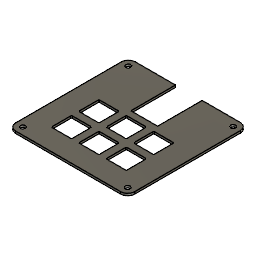
SpeedrunDeck+front (Autodesk Fusion 360 design; units mm, degrees)
part number: 2025-12-30-22-12-29-423
Autodesk Fusion 360 part; units mm, degrees
sketch "plate-2025-12-30T20_28_05.150Z" plane through (0, 0, 0) normal (0, 0, 1) x (1, 0, 0)
  line L0 (5.2708, 37.2959) -> (18.2708, 37.2959)
  line L1 (5.2708, 23.2959) -> (18.2708, 23.2959)
  line L2 (4.7708, 36.7959) -> (4.7708, 23.7959)
  line L3 (18.7708, 36.7959) -> (18.7708, 23.7959)
  arc A0 (5.2708, 37.2959) -> (4.7708, 36.7959) centre (5.2708, 36.7959) ccw
  arc A1 (18.7708, 36.7959) -> (18.2708, 37.2959) centre (18.2708, 36.7959) ccw
  arc A2 (4.7708, 23.7959) -> (5.2708, 23.2959) centre (5.2708, 23.7959) ccw
  arc A3 (18.2708, 23.2959) -> (18.7708, 23.7959) centre (18.2708, 23.7959) ccw
  line L4 (24.3208, 37.2959) -> (37.3208, 37.2959)
  line L5 (24.3208, 23.2959) -> (37.3208, 23.2959)
  line L6 (23.8208, 36.7959) -> (23.8208, 23.7959)
  line L7 (37.8208, 36.7959) -> (37.8208, 23.7959)
  arc A4 (24.3208, 37.2959) -> (23.8208, 36.7959) centre (24.3208, 36.7959) ccw
  arc A5 (37.8208, 36.7959) -> (37.3208, 37.2959) centre (37.3208, 36.7959) ccw
  arc A6 (23.8208, 23.7959) -> (24.3208, 23.2959) centre (24.3208, 23.7959) ccw
  arc A7 (37.3208, 23.2959) -> (37.8208, 23.7959) centre (37.3208, 23.7959) ccw
  line L8 (43.3708, 37.2959) -> (56.3708, 37.2959)
  line L9 (43.3708, 23.2959) -> (56.3708, 23.2959)
  line L10 (42.8708, 36.7959) -> (42.8708, 23.7959)
  line L11 (56.8708, 36.7959) -> (56.8708, 23.7959)
  arc A8 (43.3708, 37.2959) -> (42.8708, 36.7959) centre (43.3708, 36.7959) ccw
  arc A9 (56.8708, 36.7959) -> (56.3708, 37.2959) centre (56.3708, 36.7959) ccw
  arc A10 (42.8708, 23.7959) -> (43.3708, 23.2959) centre (43.3708, 23.7959) ccw
  arc A11 (56.3708, 23.2959) -> (56.8708, 23.7959) centre (56.3708, 23.7959) ccw
  line L12 (5.2708, 18.2459) -> (18.2708, 18.2459)
  line L13 (5.2708, 4.2459) -> (18.2708, 4.2459)
  line L14 (4.7708, 17.7459) -> (4.7708, 4.7459)
  line L15 (18.7708, 17.7459) -> (18.7708, 4.7459)
  arc A12 (5.2708, 18.2459) -> (4.7708, 17.7459) centre (5.2708, 17.7459) ccw
  arc A13 (18.7708, 17.7459) -> (18.2708, 18.2459) centre (18.2708, 17.7459) ccw
  arc A14 (4.7708, 4.7459) -> (5.2708, 4.2459) centre (5.2708, 4.7459) ccw
  arc A15 (18.2708, 4.2459) -> (18.7708, 4.7459) centre (18.2708, 4.7459) ccw
  line L16 (24.3208, 18.2459) -> (37.3208, 18.2459)
  line L17 (24.3208, 4.2459) -> (37.3208, 4.2459)
  line L18 (23.8208, 17.7459) -> (23.8208, 4.7459)
  line L19 (37.8208, 17.7459) -> (37.8208, 4.7459)
  arc A16 (24.3208, 18.2459) -> (23.8208, 17.7459) centre (24.3208, 17.7459) ccw
  arc A17 (37.8208, 17.7459) -> (37.3208, 18.2459) centre (37.3208, 17.7459) ccw
  arc A18 (23.8208, 4.7459) -> (24.3208, 4.2459) centre (24.3208, 4.7459) ccw
  arc A19 (37.3208, 4.2459) -> (37.8208, 4.7459) centre (37.3208, 4.7459) ccw
  line L20 (43.3708, 18.2459) -> (56.3708, 18.2459)
  line L21 (43.3708, 4.2459) -> (56.3708, 4.2459)
  line L22 (42.8708, 17.7459) -> (42.8708, 4.7459)
  line L23 (56.8708, 17.7459) -> (56.8708, 4.7459)
  arc A20 (43.3708, 18.2459) -> (42.8708, 17.7459) centre (43.3708, 17.7459) ccw
  arc A21 (56.8708, 17.7459) -> (56.3708, 18.2459) centre (56.3708, 17.7459) ccw
  arc A22 (42.8708, 4.7459) -> (43.3708, 4.2459) centre (43.3708, 4.7459) ccw
  arc A23 (56.3708, 4.2459) -> (56.8708, 4.7459) centre (56.3708, 4.7459) ccw
  line L24 (-10.2492, 72.7959) -> (72.6508, 72.7959)
  line L25 (72.6508, 72.7959) -> (72.6508, -10.6041)
  line L26 (72.6508, -10.6041) -> (-10.2492, -10.6041)
  line L27 (-10.2492, -10.6041) -> (-10.2492, 72.7959)
  line L28 (22.6008, 72.7959) -> (41.1008, 72.7959)
  line L29 (41.1008, 72.7959) -> (41.1008, 41.7959)
  line L30 (41.1008, 41.7959) -> (22.6008, 41.7959)
  line L31 (22.6008, 41.7959) -> (22.6008, 72.7959)
  circle A24 centre (-5.2492, 67.7959) radius 1.7
  circle A25 centre (-5.2492, -5.6041) radius 1.7
  circle A26 centre (67.6508, -5.6041) radius 1.7
  circle A27 centre (67.6508, 67.7959) radius 1.7
  dimension "d1" = 82.9
  dimension "d2" = 83.4
  dimension "d3" = 15.02
  dimension "d4" = 14.85
  dimension "d5" = 18.5
  dimension "d6" = 31
  dimension "d7" = 32.85
  dimension "d8" = 3.4
  dimension "d9" = 5
  dimension "d10" = 5
  dimension "d11" = 3.4
  dimension "d12" = 5
  dimension "d13" = 5
  dimension "d14" = 3.4
  dimension "d15" = 5
  dimension "d16" = 5
  dimension "d17" = 3.4
  dimension "d18" = 5
  dimension "d19" = 5
  constraint horizontal L24
  constraint vertical L25
  constraint horizontal L26
  constraint vertical L27
  constraint horizontal L28
  constraint vertical L29
  constraint horizontal L30
  constraint vertical L31
  constraint coincident L24 L28.start
  measures "d1" distance of L24.start L24.end
  measures "d2" distance of L24.end L25.end
  measures "d3" distance of L14 L27
  measures "d4" distance of L13 L26
  measures "d5" distance of L28.start L28.end
  measures "d6" distance of L28.start L30.end
  measures "d7" distance of L27 L31
  measures "d8" diameter of A24
  measures "d9" distance of L24 A24.centre
  measures "d10" distance of L27 A24.centre
  measures "d11" diameter of A25
  measures "d12" distance of L27 A25.centre
  measures "d13" distance of L26 A25.centre
  measures "d14" diameter of A26
  measures "d15" distance of L25 A26.centre
  measures "d16" distance of L26 A26.centre
  measures "d17" diameter of A27
  measures "d18" distance of L24 A27.centre
  measures "d19" distance of L25 A27.centre
extrude "Extrude1" add sketch "plate-2025-12-30T20_28_05.150Z" along normal blind 1.5 contours L24 L25 L26 L27 L29 L30 L31
fillet "Fillet1" radius 5 4 edges at (72.6508, -10.6041, 0.75) (72.6508, 72.7959, 0.75) (-10.2492, 72.7959, 0.75) (-10.2492, -10.6041, 0.75)
